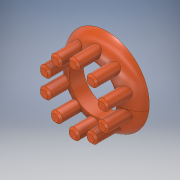
# Autodesk Inventor part: Orangatang Kegel Flat Face Adapter
Saved by Autodesk Inventor 2019.2 (Build 232265000, 265)
## iProperties
Created: 2018-11-27
Part Number: Orangatang Kegel Flat Face Adapter
Material: ABS Plastic
Document SubType Name: Modeling
Designer: Petar
Density: 1.06 g/cm^3
Appearance: Smooth - Light Orange
Author: Petar
Autodesk Inventor part; units mm, degrees
ref_plane "YZ Plane" through (0, 0, 0) normal (1, 0, 0) x (0, 1, 0)
ref_plane "XZ Plane" through (0, 0, 0) normal (0, 1, 0) x (-1, 0, 0)
ref_plane "Work Plane1" through (22.0703, 22.0585, 4.65) normal (0.1285, 0.9917, 0) x (-0.9917, 0.1285, 0)
sketch "Sketch1" plane through (22.0703, 22.0585, 4.65) normal (0.1285, 0.9917, 0) x (-0.9917, 0.1285, 0)
  line L0 (21.9945, 0) -> (-22.0404, 0) construction
  line L1 (0, -9.17) -> (0, 22.47) construction
  line L2 (-12.4923, 7.4051) -> (12.5154, 7.4051) construction
  line L3 (22.0351, 0) -> (-22.0495, 0) construction
  line L4 (-12.4923, 7.4051) -> (-12.4982, 7.4051) construction
  line L5 (-21.4921, 1.5865) -> (-22.0495, 0) construction
  spline S0 degree 4 poles (-12.4923, 7.4051) (-12.4982, 7.4051) (-12.8242, 7.3833) (-16.2631, 6.7275) (-19.5452, 4.9979) (-21.4921, 1.5865) (-22.0495, 0) knots 1 1 1 1 1 1.001686 1.104032 2 2 2 2 2
  line L6 (-19.5452, 4.9979) -> (-21.4921, 1.5865) construction
  line L7 (-12.4982, 7.4051) -> (-12.8242, 7.3833) construction
  line L8 (-12.8242, 7.3833) -> (-16.2631, 6.7275) construction
  line L9 (-16.2631, 6.7275) -> (-19.5452, 4.9979) construction
  line L10 (-22.0495, 0) -> (0, 0)
  line L11 (0, 7.4051) -> (-12.4923, 7.4051)
  line L12 (0, 7.4051) -> (0, 0)
  point P0 (19.0532, -4.65)
  constraints: 8 end point, 3 point on line, 2 collinear, 1 horizontal, 3 other
revolve "Revolution1" add sketch "Sketch1" angle 360 about axis through (22.0703, 22.0585, 4.65) along (0, 0, 1)
sketch "Sketch2" plane through (22.0703, 22.0585, 4.65) normal (0, 0, -1) x (-1, 0, 0)
  circle A0 centre (0, 0) radius 12.4923 projected
  circle A1 centre (0, -15.85) radius 2.9
  line L0 (0, -15.85) -> (0, 0) construction
  point P0 (-21.8668, -2.833)
  point P1 (22.0703, -22.0585)
  point P2 (-12.3887, -1.6051)
  dimension "d1" = 5.8
  dimension "d2" = 15.85
  constraints: 2 end point, 1 centre point, 1 vertical, 1 other
  measures "d1" diameter of A1
  measures "d2" distance of L0.start L0.end
extrude "Extrusion1" cut sketch "Sketch2" against normal through all contours A0
extrude "Extrusion2" add sketch "Sketch2" against normal blind 18 contours A1
chamfer "Chamfer1" distance 1 angle 45 1 edges at (24.9703, 6.2085, 22.65)
pattern_circular "Circular Pattern1" count 10 over 360 about axis through (22.0703, 22.0585, 4.65) along (0, 0, 1) of "Extrusion2", "Chamfer1"
body "Solid1"
